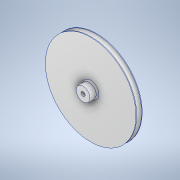
# Autodesk Inventor part: Roda
Saved by Autodesk Inventor 2021 (Build 250183000, 183)
## iProperties
Created: 2021-12-01
Part Number: Roda
Material: Alumínio 6061
Document SubType Name: Modeling
Designer: allan
Density: 2.7 g/cm^3
Appearance: Alumínio - Plano
Author: allan
Autodesk Inventor part; units mm, degrees
ref_plane "YZ Plane" through (0, 0, 0) normal (1, 0, 0) x (0, 1, 0)
ref_plane "XZ Plane" through (0, 0, 0) normal (0, 1, 0) x (-1, 0, 0)
ref_plane "XY Plane" through (0, 0, 0) normal (0, 0, 1) x (1, 0, 0)
sketch "Esboço2" plane through (0, 0, 0) normal (0, 1, 0) x (-1, 0, 0)
  line L0 (0, 0) -> (32.978, 0)
  line L1 (32.978, 0) -> (32.978, -0.5)
  line L2 (33, -3.9999) -> (33, -4.4999)
  line L3 (33, -4.4999) -> (1.5, -4.4999)
  line L4 (0, 0) -> (0, -4.4999)
  line L5 (15.5, 0) -> (18.5, 0)
  line L6 (15.5, 0) -> (14, 0)
  line L7 (17, 0) -> (18, 0)
  line L8 (17, 0) -> (23, 0)
  line L9 (0, 0) -> (1.5, 0)
  line L10 (0, 0) -> (6, 0)
  arc A0 (5, 1) -> (6, 0) centre (6.0643, 1.0643) ccw
  line L11 (5, 1) -> (5, 5.5)
  line L12 (0, 0) -> (1.5, 0)
  line L13 (0, 0) -> (1.5, 0)
  line L14 (1.5, 0) -> (1.5, 5.5)
  line L15 (5, 5.5) -> (1.5, 5.5)
  line L16 (0, 11.2552) -> (0, -29.3758)
  arc A1 (32.978, -0.5) -> (33, -3.9999) centre (32.989, -2.25) ccw
  line L17 (1.5, 0) -> (1.5, -4.4999)
  dimension "d26" = 3.5
  dimension "d27" = 33
  dimension "d45" = 6
  dimension "d48" = 4.5
  dimension "d51" = 5.5
  dimension "d52" = 0.5
  dimension "d53" = 0.5
  dimension "d54" = 1.75
  constraints: 36 end point, 6 point on line, 5 vertical, 4 horizontal, 4 point on circle, 2 centre point, 1 midpoint, 1 perpendicular
  measures "d26" distance of L1.end L2.start
  measures "d27" distance of L2.end L4.end
  measures "d45" distance of L0.start L10.end
  measures "d48" distance of L11.start L11.end
  measures "d51" distance of L9.end L14.end
  measures "d52" distance of L0.end L1.end
  measures "d53" distance of L2.start L2.end
  measures "d54" radius of A1
revolve "Revolução2" add sketch "Esboço2" angle 360 about axis through (0, 0, 11.2552) along (0, 0, -1)
